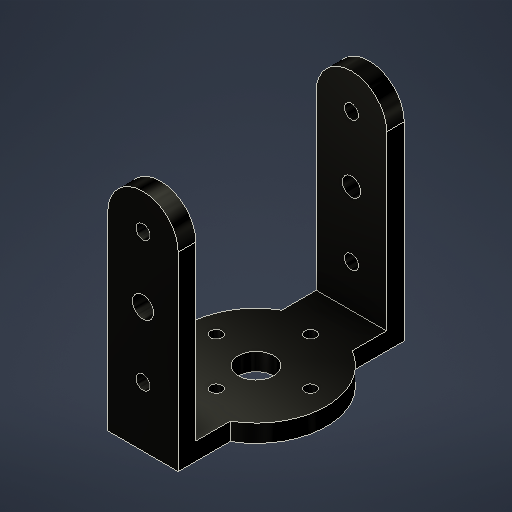
# Autodesk Inventor part: camerabracket
Saved by Autodesk Inventor 2027 (Build 310192000, 192)
## iProperties
Created: 2017-10-01
Part Number: camerabracket
Material: ABS Plastic
Document SubType Name: Modeling
Designer: david
Density: 1.06 g/cm^3
Appearance: Gunmetal
Mass: 4.77926 g
Surface Area: 38.9164 cm^2
Volume: 4.50874 cm^3
Author: david
Autodesk Inventor part; units mm, degrees
ref_plane "YZ Plane" through (0, 0, 0) normal (1, 0, 0) x (0, 1, 0)
ref_plane "XZ Plane" through (0, 0, 0) normal (0, 1, 0) x (-1, 0, 0)
ref_plane "XY Plane" through (0, 0, 0) normal (0, 0, 1) x (1, 0, 0)
sketch "Sketch1" plane through (0, 0, 0) normal (0, 0, 1) x (1, 0, 0)
  line L0 (-6.35, 0) -> (-6.35, 3.175)
  line L1 (-6.35, 3.175) -> (-6.35, 34.29)
  line L2 (6.35, 34.29) -> (6.35, 3.175)
  line L3 (6.35, 3.175) -> (6.35, 0)
  line L4 (6.35, 0) -> (-6.35, 0)
  arc A0 (6.35, 34.29) -> (-6.35, 34.29) centre (0, 34.29) ccw
  point P0 (0, 0)
  point P1 (0, 0)
  dimension "d3" = 12.7
  dimension "d4" = 40.64
  dimension "d26" = 6.35
  dimension "d27" = 3.175
  constraints: 10 end point, 2 point on circle, 2 tangent, 2 vertical, 1 centre point, 1 coincident, 1 collinear, 1 midpoint, 1 parallel, 1 perpendicular
  measures "d3" distance of L3.end L0.start
  measures "d26" radius of A0
  measures "d27" distance of L2.end L3.end
extrude "Extrusion1" add sketch "Sketch1" against normal blind 3.175
sketch "Sketch2" plane through (0, 0, -3.175) normal (0, 0, -1) x (-1, 0, 0)
  line L0 (-6.35, 34.29) -> (-6.35, 0) projected
  line L1 (6.35, 0) -> (-6.35, 0)
  line L2 (-6.35, 0) -> (-6.35, 3.175)
  line L3 (-6.35, 3.175) -> (6.35, 3.175)
  line L4 (6.35, 3.175) -> (6.35, 0)
  point P0 (0, 0)
  point P1 (-6.35, 3.175)
  dimension "d5" = 3.175
  constraints: 8 end point, 2 parallel, 1 horizontal, 1 perpendicular, 1 point on line
  measures "d5" distance between parallel lines of L1 L3
extrude "Extrusion2" add sketch "Sketch2" along normal blind 34.452
sketch "Sketch3" plane through (0, 0, -37.627) normal (0, 0, -1) x (-1, 0, 0)
  line L0 (-6.35, 0) -> (6.35, 0) projected
  line L1 (6.35, 0) -> (-6.35, 0)
  line L2 (6.35, 0) -> (6.35, 34.29)
  line L3 (-6.35, 3.175) -> (-6.35, 0) projected
  line L4 (-6.35, 0) -> (-6.35, 3.175)
  line L5 (-6.35, 3.175) -> (-6.35, 34.29)
  arc A0 (6.35, 34.29) -> (-6.35, 34.29) centre (0, 34.29) ccw
  point P0 (0, 0)
  dimension "d45" = 6.35
  dimension "d55" = 34.29
  constraints: 8 end point, 2 collinear, 2 point on circle, 2 tangent, 1 centre point, 1 perpendicular
  measures "d45" radius of A0
  measures "d55" distance of L0.end L2.end
extrude "Extrusion7" add sketch "Sketch3" along normal blind 3.175
sketch "Sketch4" plane through (-6.35, 3.175, -3.175) normal (0, 1, 0) x (1, 0, 0)
  circle A0 centre (6.35, 17.226) radius 12.7
  line L0 (0, 0) -> (0, 34.452) construction
  line L1 (0, 0) -> (12.7, 34.452) construction
  point P0 (6.35, -3.175)
  point P1 (12.7, 34.452)
  dimension "d13" = 25.4
  constraints: 2 coincident, 2 end point, 1 centre point, 1 midpoint
  measures "d13" diameter of A0
extrude "Extrusion4" add sketch "Sketch4" against normal up to surface (3.175 mm away)
sketch "Sketch6" plane through (0, 0, 0) normal (0, 0, 1) x (1, 0, 0)
  circle A0 centre (0, 34.29) radius 1.27
  circle A1 centre (0, 10.795) radius 1.27
  line L0 (0, 10.795) -> (0, 34.29) construction
  line L1 (6.35, 0) -> (-6.35, 0) construction
  line L2 (-1.27, 22.5425) -> (0, 22.5425) construction
  line L3 (-1.27, 10.795) -> (-1.27, 34.29) construction
  arc A2 (6.35, 34.29) -> (-6.35, 34.29) centre (0, 34.29) ccw projected
  line L4 (-6.35, 3.175) -> (-6.35, 34.29) construction
  line L5 (-6.35, 10.795) -> (6.35, 10.795) construction
  point P0 (0, 0)
  point P1 (0, 0)
  dimension "d18" = 2.54
  dimension "d19" = 23.495
  constraints: 8 end point, 4 midpoint, 2 horizontal alignment, 2 perpendicular, 2 point on line, 1 coincident, 1 parallel, 1 vertical, 4 other
  measures "d19" distance of L0.start L0.end
extrude "Extrusion6" cut sketch "Sketch6" against normal blind 500
sketch "Sketch8" plane through (-6.35, 3.175, -3.175) normal (0, 1, 0) x (1, 0, 0)
  circle A0 centre (6.35, 17.226) radius 3.175
  arc A1 (0, 28.2245) -> (0, 6.2275) centre (6.35, 17.226) ccw projected
  point P0 (6.35, -3.175)
  dimension "d36" = 6.35
  constraints: 1 centre point, 1 concentric
  measures "d36" diameter of A0
extrude "Extrusion9" cut sketch "Sketch8" against normal up to next
sketch "Sketch9" plane through (0, 0, 0) normal (0, 0, 1) x (1, 0, 0)
  circle A0 centre (0, 22.5425) radius 1.905
  circle A1 centre (0, 34.29) radius 1.27 construction
  circle A2 centre (0, 10.795) radius 1.27 construction
  line L0 (0, 34.29) -> (0, 10.795) construction
  point P0 (0, 0)
  point P1 (0, 22.5425)
  dimension "d39" = 3.81
  constraints: 2 end point, 1 centre point, 1 coincident, 1 midpoint, 1 vertical
  measures "d39" diameter of A0
extrude "Extrusion10" cut sketch "Sketch9" against normal up to next
sketch "Sketch10" plane through (-6.35, 3.175, -3.175) normal (0, 1, 0) x (1, 0, 0)
  circle A0 centre (6.35, 10.0521) radius 1.05 projected
  circle A1 centre (-2.159, 18.5611) radius 1.05 projected
  circle A2 centre (6.35, 27.07) radius 1.05 projected
  circle A3 centre (14.859, 18.5611) radius 1.05 projected
  point P0 (6.35, -3.175)
extrude "Extrusion11" cut sketch "Sketch10" against normal up to next
sketch "Sketch12" plane through (0, 0, -40.802) normal (0, 0, -1) x (-1, 0, 0)
  circle A0 centre (0, 22.5425) radius 1.651
  circle A1 centre (0, 22.5425) radius 1.905 projected
  point P0 (0, 0)
  dimension "d52" = 3.302
  constraints: 1 centre point, 1 concentric
  measures "d52" diameter of A0
extrude "Extrusion13" cut sketch "Sketch12" against normal up to next contours A0
body "Solid1"
